Autodesk Fusion 360 part; units mm, degrees
(part 5 of 6)
sketch "Sketch6" plane through (0, -4, 0) normal (0, -1, 0) x (1, 0, 0)
  line L0 (159.495, -1.7823) -> (159.495, -3.7827)
  line L1 (159.495, -3.7827) -> (160.296, -3.7827)
  line L2 (160.296, -3.7827) -> (160.296, -6.8819)
  line L3 (160.296, -6.8819) -> (159.495, -6.8819)
  line L4 (159.495, -6.8819) -> (159.495, -12.6821)
  line L5 (159.495, -12.6821) -> (160.296, -12.6821)
  line L6 (160.296, -12.6821) -> (160.296, -15.7827)
  line L7 (160.296, -15.7827) -> (159.495, -15.7827)
  line L8 (159.495, -15.7827) -> (159.495, -17.7817)
  line L9 (159.495, -17.7817) -> (145.496, -17.7817)
  line L10 (145.496, -17.7817) -> (145.496, -15.7827)
  line L11 (145.496, -15.7827) -> (144.695, -15.7827)
  line L12 (144.695, -15.7827) -> (144.695, -12.6821)
  line L13 (144.695, -12.6821) -> (145.496, -12.6821)
  line L14 (145.496, -12.6821) -> (145.496, -6.8819)
  line L15 (145.496, -6.8819) -> (144.695, -6.8819)
  line L16 (144.695, -6.8819) -> (144.695, -3.7827)
  line L17 (144.695, -3.7827) -> (145.496, -3.7827)
  line L18 (145.496, -3.7827) -> (145.496, -1.7823)
  line L19 (145.496, -1.7823) -> (159.495, -1.7823)
  line L20 (31.196, -3.7827) -> (31.196, -1.7823)
  line L21 (31.196, -1.7823) -> (45.1954, -1.7823)
  line L22 (45.1954, -1.7823) -> (45.1954, -3.7827)
  line L23 (45.1954, -3.7827) -> (45.9962, -3.7827)
  line L24 (45.9962, -3.7827) -> (45.9962, -6.8819)
  line L25 (45.9962, -6.8819) -> (45.1954, -6.8819)
  line L26 (45.1954, -6.8819) -> (45.1954, -12.6821)
  line L27 (45.1954, -12.6821) -> (45.9962, -12.6821)
  line L28 (45.9962, -12.6821) -> (45.9962, -15.7827)
  line L29 (45.9962, -15.7827) -> (45.1954, -15.7827)
  line L30 (45.1954, -15.7827) -> (45.1954, -17.7817)
  line L31 (45.1954, -17.7817) -> (31.196, -17.7817)
  line L32 (31.196, -17.7817) -> (31.196, -15.7827)
  line L33 (31.196, -15.7827) -> (30.3954, -15.7827)
  line L34 (30.3954, -15.7827) -> (30.3954, -12.6821)
  line L35 (30.3954, -12.6821) -> (31.196, -12.6821)
  line L36 (31.196, -12.6821) -> (31.196, -6.8819)
  line L37 (31.196, -6.8819) -> (30.3954, -6.8819)
  line L38 (30.3954, -6.8819) -> (30.3954, -3.7827)
  line L39 (30.3954, -3.7827) -> (31.196, -3.7827)
  line L40 (155.021, -36.8316) -> (155.021, -34.8327)
  line L41 (155.021, -34.8327) -> (154.22, -34.8327)
  line L42 (154.22, -34.8327) -> (154.22, -31.7321)
  line L43 (154.22, -31.7321) -> (155.021, -31.7321)
  line L44 (155.021, -31.7321) -> (155.021, -25.9319)
  line L45 (155.021, -25.9319) -> (154.22, -25.9319)
  line L46 (154.22, -25.9319) -> (154.22, -22.8327)
  line L47 (154.22, -22.8327) -> (155.021, -22.8327)
  line L48 (155.021, -22.8327) -> (155.021, -20.8323)
  line L49 (155.021, -20.8323) -> (169.02, -20.8323)
  line L50 (169.02, -20.8323) -> (169.02, -22.8327)
  line L51 (169.02, -22.8327) -> (169.821, -22.8327)
  line L52 (169.821, -22.8327) -> (169.821, -25.9319)
  line L53 (169.821, -25.9319) -> (169.02, -25.9319)
  line L54 (169.02, -25.9319) -> (169.02, -31.7321)
  line L55 (169.02, -31.7321) -> (169.821, -31.7321)
  line L56 (169.821, -31.7321) -> (169.821, -34.8327)
  line L57 (169.821, -34.8327) -> (169.02, -34.8327)
  line L58 (169.02, -34.8327) -> (169.02, -36.8316)
  line L59 (169.02, -36.8316) -> (155.021, -36.8316)
  line L60 (135.971, -36.8316) -> (135.971, -34.8327)
  line L61 (135.971, -34.8327) -> (135.17, -34.8327)
  line L62 (135.17, -34.8327) -> (135.17, -31.7321)
  line L63 (135.17, -31.7321) -> (135.971, -31.7321)
  line L64 (135.971, -31.7321) -> (135.971, -25.9319)
  line L65 (135.971, -25.9319) -> (135.17, -25.9319)
  line L66 (135.17, -25.9319) -> (135.17, -22.8327)
  line L67 (135.17, -22.8327) -> (135.971, -22.8327)
  line L68 (135.971, -22.8327) -> (135.971, -20.8323)
  line L69 (135.971, -20.8323) -> (149.97, -20.8323)
  line L70 (149.97, -20.8323) -> (149.97, -22.8327)
  line L71 (149.97, -22.8327) -> (150.771, -22.8327)
  line L72 (150.771, -22.8327) -> (150.771, -25.9319)
  line L73 (150.771, -25.9319) -> (149.97, -25.9319)
  line L74 (149.97, -25.9319) -> (149.97, -31.7321)
  line L75 (149.97, -31.7321) -> (150.771, -31.7321)
  line L76 (150.771, -31.7321) -> (150.771, -34.8327)
  line L77 (150.771, -34.8327) -> (149.97, -34.8327)
  line L78 (149.97, -34.8327) -> (149.97, -36.8316)
  line L79 (149.97, -36.8316) -> (135.971, -36.8316)
  line L80 (116.92, -36.8316) -> (116.92, -34.8327)
  line L81 (116.92, -34.8327) -> (116.119, -34.8327)
  line L82 (116.119, -34.8327) -> (116.119, -31.7321)
  line L83 (116.119, -31.7321) -> (116.92, -31.7321)
  line L84 (116.92, -31.7321) -> (116.92, -25.9319)
  line L85 (116.92, -25.9319) -> (116.119, -25.9319)
  line L86 (116.119, -25.9319) -> (116.119, -22.8327)
  line L87 (116.119, -22.8327) -> (116.92, -22.8327)
  line L88 (116.92, -22.8327) -> (116.92, -20.8323)
  line L89 (116.92, -20.8323) -> (130.92, -20.8323)
  line L90 (130.92, -20.8323) -> (130.92, -22.8327)
  line L91 (130.92, -22.8327) -> (131.721, -22.8327)
  line L92 (131.721, -22.8327) -> (131.721, -25.9319)
  line L93 (131.721, -25.9319) -> (130.92, -25.9319)
  line L94 (130.92, -25.9319) -> (130.92, -31.7321)
  line L95 (130.92, -31.7321) -> (131.721, -31.7321)
  line L96 (131.721, -31.7321) -> (131.721, -34.8327)
  line L97 (131.721, -34.8327) -> (130.92, -34.8327)
  line L98 (130.92, -34.8327) -> (130.92, -36.8316)
  line L99 (130.92, -36.8316) -> (116.92, -36.8316)
  line L100 (111.869, -20.8323) -> (111.869, -22.8327)
  line L101 (111.869, -22.8327) -> (112.67, -22.8327)
  line L102 (112.67, -22.8327) -> (112.67, -25.9319)
  line L103 (112.67, -25.9319) -> (111.869, -25.9319)
  line L104 (111.869, -25.9319) -> (111.869, -31.7321)
  line L105 (111.869, -31.7321) -> (112.67, -31.7321)
  line L106 (112.67, -31.7321) -> (112.67, -34.8327)
  line L107 (112.67, -34.8327) -> (111.869, -34.8327)
  line L108 (111.869, -34.8327) -> (111.869, -36.8316)
  line L109 (111.869, -36.8316) -> (97.8697, -36.8316)
  line L110 (97.8697, -36.8316) -> (97.8697, -34.8327)
  line L111 (97.8697, -34.8327) -> (97.0703, -34.8327)
  line L112 (97.0703, -34.8327) -> (97.0703, -31.7321)
  line L113 (97.0703, -31.7321) -> (97.8697, -31.7321)
  line L114 (97.8697, -31.7321) -> (97.8697, -25.9319)
  line L115 (97.8697, -25.9319) -> (97.0703, -25.9319)
  line L116 (97.0703, -25.9319) -> (97.0703, -22.8327)
  line L117 (97.0703, -22.8327) -> (97.8697, -22.8327)
  line L118 (97.8697, -22.8327) -> (97.8697, -20.8323)
  line L119 (97.8697, -20.8323) -> (111.869, -20.8323)
  line L120 (40.7211, -36.8316) -> (40.7211, -34.8327)
  line L121 (40.7211, -34.8327) -> (39.9203, -34.8327)
  line L122 (39.9203, -34.8327) -> (39.9203, -31.7321)
  line L123 (39.9203, -31.7321) -> (40.7211, -31.7321)
  line L124 (40.7211, -31.7321) -> (40.7211, -25.9319)
  line L125 (40.7211, -25.9319) -> (39.9203, -25.9319)
  line L126 (39.9203, -25.9319) -> (39.9203, -22.8327)
  line L127 (39.9203, -22.8327) -> (40.7211, -22.8327)
  line L128 (40.7211, -22.8327) -> (40.7211, -20.8323)
  line L129 (40.7211, -20.8323) -> (54.7204, -20.8323)
  line L130 (54.7204, -20.8323) -> (54.7204, -22.8327)
  line L131 (54.7204, -22.8327) -> (55.5212, -22.8327)
  line L132 (55.5212, -22.8327) -> (55.5212, -25.9319)
  line L133 (55.5212, -25.9319) -> (54.7204, -25.9319)
  line L134 (54.7204, -25.9319) -> (54.7204, -31.7321)
  line L135 (54.7204, -31.7321) -> (55.5212, -31.7321)
  line L136 (55.5212, -31.7321) -> (55.5212, -34.8327)
  line L137 (55.5212, -34.8327) -> (54.7204, -34.8327)
  line L138 (54.7204, -34.8327) -> (54.7204, -36.8316)
  line L139 (54.7204, -36.8316) -> (40.7211, -36.8316)
  line L140 (35.6704, -20.8323) -> (35.6704, -22.8327)
  line L141 (35.6704, -22.8327) -> (36.4712, -22.8327)
  line L142 (36.4712, -22.8327) -> (36.4712, -25.9319)
  line L143 (36.4712, -25.9319) -> (35.6704, -25.9319)
  line L144 (35.6704, -25.9319) -> (35.6704, -31.7321)
  line L145 (35.6704, -31.7321) -> (36.4712, -31.7321)
  line L146 (36.4712, -31.7321) -> (36.4712, -34.8327)
  line L147 (36.4712, -34.8327) -> (35.6704, -34.8327)
  line L148 (35.6704, -34.8327) -> (35.6704, -36.8316)
  line L149 (35.6704, -36.8316) -> (21.671, -36.8316)
  line L150 (21.671, -36.8316) -> (21.671, -34.8327)
  line L151 (21.671, -34.8327) -> (20.8704, -34.8327)
  line L152 (20.8704, -34.8327) -> (20.8704, -31.7321)
  line L153 (20.8704, -31.7321) -> (21.671, -31.7321)
  line L154 (21.671, -31.7321) -> (21.671, -25.9319)
  line L155 (21.671, -25.9319) -> (20.8704, -25.9319)
  line L156 (20.8704, -25.9319) -> (20.8704, -22.8327)
  line L157 (20.8704, -22.8327) -> (21.671, -22.8327)
  line L158 (21.671, -22.8327) -> (21.671, -20.8323)
  line L159 (21.671, -20.8323) -> (35.6704, -20.8323)
  line L160 (155.021, -55.8816) -> (155.021, -53.8826)
  line L161 (155.021, -53.8826) -> (154.22, -53.8826)
  line L162 (154.22, -53.8826) -> (154.22, -50.782)
  line L163 (154.22, -50.782) -> (155.021, -50.782)
  line L164 (155.021, -50.782) -> (155.021, -44.982)
  line L165 (155.021, -44.982) -> (154.22, -44.982)
  line L166 (154.22, -44.982) -> (154.22, -41.8828)
  line L167 (154.22, -41.8828) -> (155.021, -41.8828)
  line L168 (155.021, -41.8828) -> (155.021, -39.8824)
  line L169 (155.021, -39.8824) -> (169.02, -39.8824)
  line L170 (169.02, -39.8824) -> (169.02, -41.8828)
  line L171 (169.02, -41.8828) -> (169.821, -41.8828)
  line L172 (169.821, -41.8828) -> (169.821, -44.982)
  line L173 (169.821, -44.982) -> (169.02, -44.982)
  line L174 (169.02, -44.982) -> (169.02, -50.782)
  line L175 (169.02, -50.782) -> (169.821, -50.782)
  line L176 (169.821, -50.782) -> (169.821, -53.8826)
  line L177 (169.821, -53.8826) -> (169.02, -53.8826)
  line L178 (169.02, -53.8826) -> (169.02, -55.8816)
  line L179 (169.02, -55.8816) -> (155.021, -55.8816)
  line L180 (16.6205, -20.8323) -> (16.6205, -22.8327)
  line L181 (16.6205, -22.8327) -> (17.4212, -22.8327)
  line L182 (17.4212, -22.8327) -> (17.4212, -25.9319)
  line L183 (17.4212, -25.9319) -> (16.6205, -25.9319)
  line L184 (16.6205, -25.9319) -> (16.6205, -31.7321)
  line L185 (16.6205, -31.7321) -> (17.4212, -31.7321)
  line L186 (17.4212, -31.7321) -> (17.4212, -34.8327)
  line L187 (17.4212, -34.8327) -> (16.6205, -34.8327)
  line L188 (16.6205, -34.8327) -> (16.6205, -36.8316)
  line L189 (16.6205, -36.8316) -> (2.621, -36.8316)
  line L190 (2.621, -36.8316) -> (2.621, -34.8327)
  line L191 (2.621, -34.8327) -> (1.8204, -34.8327)
  line L192 (1.8204, -34.8327) -> (1.8204, -31.7321)
  line L193 (1.8204, -31.7321) -> (2.621, -31.7321)
  line L194 (2.621, -31.7321) -> (2.621, -25.9319)
  line L195 (2.621, -25.9319) -> (1.8204, -25.9319)
  line L196 (1.8204, -25.9319) -> (1.8204, -22.8327)
  line L197 (1.8204, -22.8327) -> (2.621, -22.8327)
  line L198 (2.621, -22.8327) -> (2.621, -20.8323)
  line L199 (2.621, -20.8323) -> (16.6205, -20.8323)
  line L200 (21.671, -55.8816) -> (21.671, -53.8826)
  line L201 (21.671, -53.8826) -> (20.8704, -53.8826)
  line L202 (20.8704, -53.8826) -> (20.8704, -50.782)
  line L203 (20.8704, -50.782) -> (21.671, -50.782)
  line L204 (21.671, -50.782) -> (21.671, -44.982)
  line L205 (21.671, -44.982) -> (20.8704, -44.982)
  line L206 (20.8704, -44.982) -> (20.8704, -41.8828)
  line L207 (20.8704, -41.8828) -> (21.671, -41.8828)
  line L208 (21.671, -41.8828) -> (21.671, -39.8824)
  line L209 (21.671, -39.8824) -> (35.6704, -39.8824)
  line L210 (35.6704, -39.8824) -> (35.6704, -41.8828)
  line L211 (35.6704, -41.8828) -> (36.4712, -41.8828)
  line L212 (36.4712, -41.8828) -> (36.4712, -44.982)
  line L213 (36.4712, -44.982) -> (35.6704, -44.982)
  line L214 (35.6704, -44.982) -> (35.6704, -50.782)
  line L215 (35.6704, -50.782) -> (36.4712, -50.782)
  line L216 (36.4712, -50.782) -> (36.4712, -53.8826)
  line L217 (36.4712, -53.8826) -> (35.6704, -53.8826)
  line L218 (35.6704, -53.8826) -> (35.6704, -55.8816)
  line L219 (35.6704, -55.8816) -> (21.671, -55.8816)
  line L220 (97.8697, -55.8816) -> (97.8697, -53.8826)
  line L221 (97.8697, -53.8826) -> (97.0703, -53.8826)
  line L222 (97.0703, -53.8826) -> (97.0703, -50.782)
  line L223 (97.0703, -50.782) -> (97.8697, -50.782)
  line L224 (97.8697, -50.782) -> (97.8697, -44.982)
  line L225 (97.8697, -44.982) -> (97.0703, -44.982)
  line L226 (97.0703, -44.982) -> (97.0703, -41.8828)
  line L227 (97.0703, -41.8828) -> (97.8697, -41.8828)
  line L228 (97.8697, -41.8828) -> (97.8697, -39.8824)
  line L229 (97.8697, -39.8824) -> (111.869, -39.8824)
  line L230 (111.869, -39.8824) -> (111.869, -41.8828)
  line L231 (111.869, -41.8828) -> (112.67, -41.8828)
  line L232 (112.67, -41.8828) -> (112.67, -44.982)
  line L233 (112.67, -44.982) -> (111.869, -44.982)
  line L234 (111.869, -44.982) -> (111.869, -50.782)
  line L235 (111.869, -50.782) -> (112.67, -50.782)
  line L236 (112.67, -50.782) -> (112.67, -53.8826)
  line L237 (112.67, -53.8826) -> (111.869, -53.8826)
  line L238 (111.869, -53.8826) -> (111.869, -55.8816)
  line L239 (111.869, -55.8816) -> (97.8697, -55.8816)
  line L240 (54.7204, -39.8824) -> (54.7204, -41.8828)
  line L241 (54.7204, -41.8828) -> (55.5212, -41.8828)
  line L242 (55.5212, -41.8828) -> (55.5212, -44.982)
  line L243 (55.5212, -44.982) -> (54.7204, -44.982)
  line L244 (54.7204, -44.982) -> (54.7204, -50.782)
  line L245 (54.7204, -50.782) -> (55.5212, -50.782)
  line L246 (55.5212, -50.782) -> (55.5212, -53.8826)
  line L247 (55.5212, -53.8826) -> (54.7204, -53.8826)
  line L248 (54.7204, -53.8826) -> (54.7204, -55.8816)
  line L249 (54.7204, -55.8816) -> (40.7211, -55.8816)
  line L250 (40.7211, -55.8816) -> (40.7211, -53.8826)
  line L251 (40.7211, -53.8826) -> (39.9203, -53.8826)
  line L252 (39.9203, -53.8826) -> (39.9203, -50.782)
  line L253 (39.9203, -50.782) -> (40.7211, -50.782)
  line L254 (40.7211, -50.782) -> (40.7211, -44.982)
  line L255 (40.7211, -44.982) -> (39.9203, -44.982)
  line L256 (39.9203, -44.982) -> (39.9203, -41.8828)
  line L257 (39.9203, -41.8828) -> (40.7211, -41.8828)
  line L258 (40.7211, -41.8828) -> (40.7211, -39.8824)
  line L259 (40.7211, -39.8824) -> (54.7204, -39.8824)
  line L260 (92.8204, -20.8323) -> (92.8204, -22.8327)
  line L261 (92.8204, -22.8327) -> (93.6198, -22.8327)
  line L262 (93.6198, -22.8327) -> (93.6198, -25.9319)
  line L263 (93.6198, -25.9319) -> (92.8204, -25.9319)
  line L264 (92.8204, -25.9319) -> (92.8204, -31.7321)
  line L265 (92.8204, -31.7321) -> (93.6198, -31.7321)
  line L266 (93.6198, -31.7321) -> (93.6198, -34.8327)
  line L267 (93.6198, -34.8327) -> (92.8204, -34.8327)
  line L268 (92.8204, -34.8327) -> (92.8204, -36.8316)
  line L269 (92.8204, -36.8316) -> (78.8211, -36.8316)
  line L270 (78.8211, -36.8316) -> (78.8211, -34.8327)
  line L271 (78.8211, -34.8327) -> (78.0203, -34.8327)
  line L272 (78.0203, -34.8327) -> (78.0203, -31.7321)
  line L273 (78.0203, -31.7321) -> (78.8211, -31.7321)
  line L274 (78.8211, -31.7321) -> (78.8211, -25.9319)
  line L275 (78.8211, -25.9319) -> (78.0203, -25.9319)
  line L276 (78.0203, -25.9319) -> (78.0203, -22.8327)
  line L277 (78.0203, -22.8327) -> (78.8211, -22.8327)
  line L278 (78.8211, -22.8327) -> (78.8211, -20.8323)
  line L279 (78.8211, -20.8323) -> (92.8204, -20.8323)
  line L280 (130.92, -39.8824) -> (130.92, -41.8828)
  line L281 (130.92, -41.8828) -> (131.721, -41.8828)
  line L282 (131.721, -41.8828) -> (131.721, -44.982)
  line L283 (131.721, -44.982) -> (130.92, -44.982)
  line L284 (130.92, -44.982) -> (130.92, -50.782)
  line L285 (130.92, -50.782) -> (131.721, -50.782)
  line L286 (131.721, -50.782) -> (131.721, -53.8826)
  line L287 (131.721, -53.8826) -> (130.92, -53.8826)
  line L288 (130.92, -53.8826) -> (130.92, -55.8816)
  line L289 (130.92, -55.8816) -> (116.92, -55.8816)
  line L290 (116.92, -55.8816) -> (116.92, -53.8826)
  line L291 (116.92, -53.8826) -> (116.119, -53.8826)
  line L292 (116.119, -53.8826) -> (116.119, -50.782)
  line L293 (116.119, -50.782) -> (116.92, -50.782)
  line L294 (116.92, -50.782) -> (116.92, -44.982)
  line L295 (116.92, -44.982) -> (116.119, -44.982)
  line L296 (116.119, -44.982) -> (116.119, -41.8828)
  line L297 (116.119, -41.8828) -> (116.92, -41.8828)
  line L298 (116.92, -41.8828) -> (116.92, -39.8824)
  line L299 (116.92, -39.8824) -> (130.92, -39.8824)
  line L300 (188.07, -20.8323) -> (188.07, -22.8327)
  line L301 (188.07, -22.8327) -> (188.871, -22.8327)
  line L302 (188.871, -22.8327) -> (188.871, -25.9319)
  line L303 (188.871, -25.9319) -> (188.07, -25.9319)
  line L304 (188.07, -25.9319) -> (188.07, -31.7321)
  line L305 (188.07, -31.7321) -> (188.871, -31.7321)
  line L306 (188.871, -31.7321) -> (188.871, -34.8327)
  line L307 (188.871, -34.8327) -> (188.07, -34.8327)
  line L308 (188.07, -34.8327) -> (188.07, -36.8316)
  line L309 (188.07, -36.8316) -> (174.071, -36.8316)
  line L310 (174.071, -36.8316) -> (174.071, -34.8327)
  line L311 (174.071, -34.8327) -> (173.27, -34.8327)
  line L312 (173.27, -34.8327) -> (173.27, -31.7321)
  line L313 (173.27, -31.7321) -> (174.071, -31.7321)
  line L314 (174.071, -31.7321) -> (174.071, -25.9319)
  line L315 (174.071, -25.9319) -> (173.27, -25.9319)
  line L316 (173.27, -25.9319) -> (173.27, -22.8327)
  line L317 (173.27, -22.8327) -> (174.071, -22.8327)
  line L318 (174.071, -22.8327) -> (174.071, -20.8323)
  line L319 (174.071, -20.8323) -> (188.07, -20.8323)
  line L320 (69.2961, -17.7817) -> (69.2961, -15.7827)
  line L321 (69.2961, -15.7827) -> (68.4953, -15.7827)
  line L322 (68.4953, -15.7827) -> (68.4953, -12.6821)
  line L323 (68.4953, -12.6821) -> (69.2961, -12.6821)
  line L324 (69.2961, -12.6821) -> (69.2961, -6.8819)
  line L325 (69.2961, -6.8819) -> (68.4953, -6.8819)
  line L326 (68.4953, -6.8819) -> (68.4953, -3.7827)
  line L327 (68.4953, -3.7827) -> (69.2961, -3.7827)
  line L328 (69.2961, -3.7827) -> (69.2961, -1.7823)
  line L329 (69.2961, -1.7823) -> (83.2954, -1.7823)
  line L330 (83.2954, -1.7823) -> (83.2954, -3.7827)
  line L331 (83.2954, -3.7827) -> (84.0962, -3.7827)
  line L332 (84.0962, -3.7827) -> (84.0962, -6.8819)
  line L333 (84.0962, -6.8819) -> (83.2954, -6.8819)
  line L334 (83.2954, -6.8819) -> (83.2954, -12.6821)
  line L335 (83.2954, -12.6821) -> (84.0962, -12.6821)
  line L336 (84.0962, -12.6821) -> (84.0962, -15.7827)
  line L337 (84.0962, -15.7827) -> (83.2954, -15.7827)
  line L338 (83.2954, -15.7827) -> (83.2954, -17.7817)
  line L339 (83.2954, -17.7817) -> (69.2961, -17.7817)
  line L340 (164.546, -17.7817) -> (164.546, -15.7827)
  line L341 (164.546, -15.7827) -> (163.745, -15.7827)
  line L342 (163.745, -15.7827) -> (163.745, -12.6821)
  line L343 (163.745, -12.6821) -> (164.546, -12.6821)
  line L344 (164.546, -12.6821) -> (164.546, -6.8819)
  line L345 (164.546, -6.8819) -> (163.745, -6.8819)
  line L346 (163.745, -6.8819) -> (163.745, -3.7827)
  line L347 (163.745, -3.7827) -> (164.546, -3.7827)
  line L348 (164.546, -3.7827) -> (164.546, -1.7823)
  line L349 (164.546, -1.7823) -> (178.545, -1.7823)
  line L350 (178.545, -1.7823) -> (178.545, -3.7827)
  line L351 (178.545, -3.7827) -> (179.346, -3.7827)
  line L352 (179.346, -3.7827) -> (179.346, -6.8819)
  line L353 (179.346, -6.8819) -> (178.545, -6.8819)
  line L354 (178.545, -6.8819) -> (178.545, -12.6821)
  line L355 (178.545, -12.6821) -> (179.346, -12.6821)
  line L356 (179.346, -12.6821) -> (179.346, -15.7827)
  line L357 (179.346, -15.7827) -> (178.545, -15.7827)
  line L358 (178.545, -15.7827) -> (178.545, -17.7817)
  line L359 (178.545, -17.7817) -> (164.546, -17.7817)
  line L360 (64.2454, -1.7823) -> (64.2454, -3.7827)
  line L361 (64.2454, -3.7827) -> (65.0462, -3.7827)
  line L362 (65.0462, -3.7827) -> (65.0462, -6.8819)
  line L363 (65.0462, -6.8819) -> (64.2454, -6.8819)
  line L364 (64.2454, -6.8819) -> (64.2454, -12.6821)
  line L365 (64.2454, -12.6821) -> (65.0462, -12.6821)
  line L366 (65.0462, -12.6821) -> (65.0462, -15.7827)
  line L367 (65.0462, -15.7827) -> (64.2454, -15.7827)
  line L368 (64.2454, -15.7827) -> (64.2454, -17.7817)
  line L369 (64.2454, -17.7817) -> (50.2461, -17.7817)
  line L370 (50.2461, -17.7817) -> (50.2461, -15.7827)
  line L371 (50.2461, -15.7827) -> (49.4453, -15.7827)
  line L372 (49.4453, -15.7827) -> (49.4453, -12.6821)
  line L373 (49.4453, -12.6821) -> (50.2461, -12.6821)
  line L374 (50.2461, -12.6821) -> (50.2461, -6.8819)
  line L375 (50.2461, -6.8819) -> (49.4453, -6.8819)
  line L376 (49.4453, -6.8819) -> (49.4453, -3.7827)
  line L377 (49.4453, -3.7827) -> (50.2461, -3.7827)
  line L378 (50.2461, -3.7827) -> (50.2461, -1.7823)
  line L379 (50.2461, -1.7823) -> (64.2454, -1.7823)
  line L380 (126.446, -3.7827) -> (126.446, -1.7823)
  line L381 (126.446, -1.7823) -> (140.445, -1.7823)
  line L382 (140.445, -1.7823) -> (140.445, -3.7827)
  line L383 (140.445, -3.7827) -> (141.246, -3.7827)
  line L384 (141.246, -3.7827) -> (141.246, -6.8819)
  line L385 (141.246, -6.8819) -> (140.445, -6.8819)
  line L386 (140.445, -6.8819) -> (140.445, -12.6821)
  line L387 (140.445, -12.6821) -> (141.246, -12.6821)
  line L388 (141.246, -12.6821) -> (141.246, -15.7827)
  line L389 (141.246, -15.7827) -> (140.445, -15.7827)
  line L390 (140.445, -15.7827) -> (140.445, -17.7817)
  line L391 (140.445, -17.7817) -> (126.446, -17.7817)
  line L392 (126.446, -17.7817) -> (126.446, -15.7827)
  line L393 (126.446, -15.7827) -> (125.645, -15.7827)
  line L394 (125.645, -15.7827) -> (125.645, -12.6821)
  line L395 (125.645, -12.6821) -> (126.446, -12.6821)
  line L396 (126.446, -12.6821) -> (126.446, -6.8819)
  line L397 (126.446, -6.8819) -> (125.645, -6.8819)
  line L398 (125.645, -6.8819) -> (125.645, -3.7827)
  line L399 (125.645, -3.7827) -> (126.446, -3.7827)
  line L400 (92.8204, -53.8826) -> (92.8204, -55.8816)
  line L401 (92.8204, -55.8816) -> (78.8211, -55.8816)
  line L402 (78.8211, -55.8816) -> (78.8211, -53.8826)
  line L403 (78.8211, -53.8826) -> (78.0203, -53.8826)
  line L404 (78.0203, -53.8826) -> (78.0203, -50.782)
  line L405 (78.0203, -50.782) -> (78.8211, -50.782)
  line L406 (78.8211, -50.782) -> (78.8211, -44.982)
  line L407 (78.8211, -44.982) -> (78.0203, -44.982)
  line L408 (78.0203, -44.982) -> (78.0203, -41.8828)
  line L409 (78.0203, -41.8828) -> (78.8211, -41.8828)
  line L410 (78.8211, -41.8828) -> (78.8211, -39.8824)
  line L411 (78.8211, -39.8824) -> (92.8204, -39.8824)
  line L412 (92.8204, -39.8824) -> (92.8204, -41.8828)
  line L413 (92.8204, -41.8828) -> (93.6198, -41.8828)
  line L414 (93.6198, -41.8828) -> (93.6198, -44.982)
  line L415 (93.6198, -44.982) -> (92.8204, -44.982)
  line L416 (92.8204, -44.982) -> (92.8204, -50.782)
  line L417 (92.8204, -50.782) -> (93.6198, -50.782)
  line L418 (93.6198, -50.782) -> (93.6198, -53.8826)
  line L419 (93.6198, -53.8826) -> (92.8204, -53.8826)
  line L420 (135.971, -41.8828) -> (135.971, -39.8824)
  line L421 (135.971, -39.8824) -> (149.97, -39.8824)
  line L422 (149.97, -39.8824) -> (149.97, -41.8828)
  line L423 (149.97, -41.8828) -> (150.771, -41.8828)
  line L424 (150.771, -41.8828) -> (150.771, -44.982)
  line L425 (150.771, -44.982) -> (149.97, -44.982)
  line L426 (149.97, -44.982) -> (149.97, -50.782)
  line L427 (149.97, -50.782) -> (150.771, -50.782)
  line L428 (150.771, -50.782) -> (150.771, -53.8826)
  line L429 (150.771, -53.8826) -> (149.97, -53.8826)
  line L430 (149.97, -53.8826) -> (149.97, -55.8816)
  line L431 (149.97, -55.8816) -> (135.971, -55.8816)
  line L432 (135.971, -55.8816) -> (135.971, -53.8826)
  line L433 (135.971, -53.8826) -> (135.17, -53.8826)
  line L434 (135.17, -53.8826) -> (135.17, -50.782)
  line L435 (135.17, -50.782) -> (135.971, -50.782)
  line L436 (135.971, -50.782) -> (135.971, -44.982)
  line L437 (135.971, -44.982) -> (135.17, -44.982)
  line L438 (135.17, -44.982) -> (135.17, -41.8828)
  line L439 (135.17, -41.8828) -> (135.971, -41.8828)
  line L440 (59.7711, -41.8828) -> (59.7711, -39.8824)
  line L441 (59.7711, -39.8824) -> (73.7704, -39.8824)
  line L442 (73.7704, -39.8824) -> (73.7704, -41.8828)
  line L443 (73.7704, -41.8828) -> (74.5712, -41.8828)
  line L444 (74.5712, -41.8828) -> (74.5712, -44.982)
  line L445 (74.5712, -44.982) -> (73.7704, -44.982)
  line L446 (73.7704, -44.982) -> (73.7704, -50.782)
  line L447 (73.7704, -50.782) -> (74.5712, -50.782)
  line L448 (74.5712, -50.782) -> (74.5712, -53.8826)
  line L449 (74.5712, -53.8826) -> (73.7704, -53.8826)
  line L450 (73.7704, -53.8826) -> (73.7704, -55.8816)
  line L451 (73.7704, -55.8816) -> (59.7711, -55.8816)
  line L452 (59.7711, -55.8816) -> (59.7711, -53.8826)
  line L453 (59.7711, -53.8826) -> (58.9703, -53.8826)
  line L454 (58.9703, -53.8826) -> (58.9703, -50.782)
  line L455 (58.9703, -50.782) -> (59.7711, -50.782)
  line L456 (59.7711, -50.782) -> (59.7711, -44.982)
  line L457 (59.7711, -44.982) -> (58.9703, -44.982)
  line L458 (58.9703, -44.982) -> (58.9703, -41.8828)
  line L459 (58.9703, -41.8828) -> (59.7711, -41.8828)
  line L460 (16.6205, -53.8826) -> (16.6205, -55.8816)
  line L461 (16.6205, -55.8816) -> (2.621, -55.8816)
  line L462 (2.621, -55.8816) -> (2.621, -53.8826)
  line L463 (2.621, -53.8826) -> (1.8204, -53.8826)
  line L464 (1.8204, -53.8826) -> (1.8204, -50.782)
  line L465 (1.8204, -50.782) -> (2.621, -50.782)
  line L466 (2.621, -50.782) -> (2.621, -44.982)
  line L467 (2.621, -44.982) -> (1.8204, -44.982)
  line L468 (1.8204, -44.982) -> (1.8204, -41.8828)
  line L469 (1.8204, -41.8828) -> (2.621, -41.8828)
  line L470 (2.621, -41.8828) -> (2.621, -39.8824)
  line L471 (2.621, -39.8824) -> (16.6205, -39.8824)
  line L472 (16.6205, -39.8824) -> (16.6205, -41.8828)
  line L473 (16.6205, -41.8828) -> (17.4212, -41.8828)
  line L474 (17.4212, -41.8828) -> (17.4212, -44.982)
  line L475 (17.4212, -44.982) -> (16.6205, -44.982)
  line L476 (16.6205, -44.982) -> (16.6205, -50.782)
  line L477 (16.6205, -50.782) -> (17.4212, -50.782)
  line L478 (17.4212, -50.782) -> (17.4212, -53.8826)
  line L479 (17.4212, -53.8826) -> (16.6205, -53.8826)
  line L480 (174.071, -41.8828) -> (174.071, -39.8824)
  line L481 (174.071, -39.8824) -> (188.07, -39.8824)
  line L482 (188.07, -39.8824) -> (188.07, -41.8828)
  line L483 (188.07, -41.8828) -> (188.871, -41.8828)
  line L484 (188.871, -41.8828) -> (188.871, -44.982)
  line L485 (188.871, -44.982) -> (188.07, -44.982)
  line L486 (188.07, -44.982) -> (188.07, -50.782)
  line L487 (188.07, -50.782) -> (188.871, -50.782)
  line L488 (188.871, -50.782) -> (188.871, -53.8826)
  line L489 (188.871, -53.8826) -> (188.07, -53.8826)
  line L490 (188.07, -53.8826) -> (188.07, -55.8816)
  line L491 (188.07, -55.8816) -> (174.071, -55.8816)
  line L492 (174.071, -55.8816) -> (174.071, -53.8826)
  line L493 (174.071, -53.8826) -> (173.27, -53.8826)
  line L494 (173.27, -53.8826) -> (173.27, -50.782)
  line L495 (173.27, -50.782) -> (174.071, -50.782)
  line L496 (174.071, -50.782) -> (174.071, -44.982)
  line L497 (174.071, -44.982) -> (173.27, -44.982)
  line L498 (173.27, -44.982) -> (173.27, -41.8828)
  line L499 (173.27, -41.8828) -> (174.071, -41.8828)
  line L500 (73.7704, -34.8327) -> (73.7704, -36.8316)
  line L501 (73.7704, -36.8316) -> (59.7711, -36.8316)
  line L502 (59.7711, -36.8316) -> (59.7711, -34.8327)
  line L503 (59.7711, -34.8327) -> (58.9703, -34.8327)
  line L504 (58.9703, -34.8327) -> (58.9703, -31.7321)
  line L505 (58.9703, -31.7321) -> (59.7711, -31.7321)
  line L506 (59.7711, -31.7321) -> (59.7711, -25.9319)
  line L507 (59.7711, -25.9319) -> (58.9703, -25.9319)
  line L508 (58.9703, -25.9319) -> (58.9703, -22.8327)
  line L509 (58.9703, -22.8327) -> (59.7711, -22.8327)
  line L510 (59.7711, -22.8327) -> (59.7711, -20.8323)
  line L511 (59.7711, -20.8323) -> (73.7704, -20.8323)
  line L512 (73.7704, -20.8323) -> (73.7704, -22.8327)
  line L513 (73.7704, -22.8327) -> (74.5712, -22.8327)
  line L514 (74.5712, -22.8327) -> (74.5712, -25.9319)
  line L515 (74.5712, -25.9319) -> (73.7704, -25.9319)
  line L516 (73.7704, -25.9319) -> (73.7704, -31.7321)
  line L517 (73.7704, -31.7321) -> (74.5712, -31.7321)
  line L518 (74.5712, -31.7321) -> (74.5712, -34.8327)
  line L519 (74.5712, -34.8327) -> (73.7704, -34.8327)
  line L520 (26.1455, -15.7827) -> (26.1455, -17.7817)
  line L521 (26.1455, -17.7817) -> (12.146, -17.7817)
  line L522 (12.146, -17.7817) -> (12.146, -15.7827)
  line L523 (12.146, -15.7827) -> (11.3454, -15.7827)
  line L524 (11.3454, -15.7827) -> (11.3454, -12.6821)
  line L525 (11.3454, -12.6821) -> (12.146, -12.6821)
  line L526 (12.146, -12.6821) -> (12.146, -6.8819)
  line L527 (12.146, -6.8819) -> (11.3454, -6.8819)
  line L528 (11.3454, -6.8819) -> (11.3454, -3.7827)
  line L529 (11.3454, -3.7827) -> (12.146, -3.7827)
  line L530 (12.146, -3.7827) -> (12.146, -1.7823)
  line L531 (12.146, -1.7823) -> (26.1455, -1.7823)
  line L532 (26.1455, -1.7823) -> (26.1455, -3.7827)
  line L533 (26.1455, -3.7827) -> (26.9462, -3.7827)
  line L534 (26.9462, -3.7827) -> (26.9462, -6.8819)
  line L535 (26.9462, -6.8819) -> (26.1455, -6.8819)
  line L536 (26.1455, -6.8819) -> (26.1455, -12.6821)
  line L537 (26.1455, -12.6821) -> (26.9462, -12.6821)
  line L538 (26.9462, -12.6821) -> (26.9462, -15.7827)
  line L539 (26.9462, -15.7827) -> (26.1455, -15.7827)
  arc A0 (190.596, -18.7817) -> (188.596, -16.7817) centre (188.596, -18.7817) ccw
  line L540 (188.596, -16.7817) -> (184.846, -16.7817)
  arc A1 (182.846, -14.7817) -> (184.846, -16.7817) centre (184.846, -14.7817) ccw
  line L541 (182.846, -14.7817) -> (182.846, -2.2564)
  arc A2 (182.846, -2.2564) -> (180.846, -0.2564) centre (180.846, -2.2564) ccw
  line L542 (180.846, -0.2564) -> (167.0351, -0.2565)
  arc A3 (9.8454, -0.2576) -> (7.8454, -2.2576) centre (9.8454, -2.2576) ccw
  line L543 (7.8454, -2.2576) -> (7.8454, -14.7817)
  arc A4 (5.8454, -16.7817) -> (7.8454, -14.7817) centre (5.8454, -14.7817) ccw
  line L544 (5.8454, -16.7817) -> (2.0951, -16.7817)
  arc A5 (2.0951, -16.7817) -> (0.0951, -18.7817) centre (2.0951, -18.7817) ccw
  line L545 (0.0951, -18.7817) -> (0.0951, -55.4069)
  line L546 (0.0951, -55.4069) -> (0.102, -55.5639)
  line L547 (0.102, -55.5639) -> (0.1199, -55.7209)
  line L548 (0.1199, -55.7209) -> (0.1502, -55.874)
  line L549 (0.1502, -55.874) -> (0.1929, -56.0268)
  line L550 (0.1929, -56.0268) -> (0.248, -56.1728)
  line L551 (0.248, -56.1728) -> (0.3128, -56.315)
  line L552 (0.3128, -56.315) -> (0.39, -56.4526)
  line L553 (0.39, -56.4526) -> (0.4768, -56.5838)
  line L554 (0.4768, -56.5838) -> (0.5746, -56.7062)
  line L555 (0.5746, -56.7062) -> (0.6808, -56.8219)
  line L556 (0.6808, -56.8219) -> (0.7965, -56.9281)
  line L557 (0.7965, -56.9281) -> (0.9192, -57.0258)
  line L558 (0.9192, -57.0258) -> (1.0501, -57.113)
  line L559 (1.0501, -57.113) -> (1.1879, -57.1899)
  line L560 (1.1879, -57.1899) -> (1.3298, -57.2548)
  line L561 (1.3298, -57.2548) -> (1.4759, -57.3098)
  line L562 (1.4759, -57.3098) -> (1.6288, -57.3525)
  line L563 (1.6288, -57.3525) -> (1.7818, -57.3828)
  line L564 (1.7818, -57.3828) -> (1.9389, -57.4008)
  line L565 (1.9389, -57.4008) -> (2.096, -57.4075)
  line L566 (2.096, -57.4075) -> (6.5216, -57.4075)
  line L567 (188.597, -57.4075) -> (188.753, -57.4008)
  line L568 (188.753, -57.4008) -> (188.908, -57.3828)
  line L569 (188.908, -57.3828) -> (189.063, -57.3525)
  line L570 (189.063, -57.3525) -> (189.214, -57.3098)
  line L571 (189.214, -57.3098) -> (189.362, -57.2548)
  line L572 (189.362, -57.2548) -> (189.504, -57.1899)
  line L573 (189.504, -57.1899) -> (189.64, -57.113)
  line L574 (189.64, -57.113) -> (189.771, -57.0258)
  line L575 (189.771, -57.0258) -> (189.895, -56.9281)
  line L576 (189.895, -56.9281) -> (190.011, -56.8219)
  line L577 (190.011, -56.8219) -> (190.117, -56.7062)
  line L578 (190.117, -56.7062) -> (190.215, -56.5838)
  line L579 (190.215, -56.5838) -> (190.302, -56.4526)
  line L580 (190.302, -56.4526) -> (190.379, -56.315)
  line L581 (190.379, -56.315) -> (190.444, -56.1728)
  line L582 (190.444, -56.1728) -> (190.499, -56.0268)
  line L583 (190.499, -56.0268) -> (190.54, -55.874)
  line L584 (190.54, -55.874) -> (190.572, -55.7209)
  line L585 (190.572, -55.7209) -> (190.59, -55.5639)
  line L586 (190.59, -55.5639) -> (190.596, -55.4069)
  line L587 (190.596, -55.4069) -> (190.596, -18.7817)
  line L588 (97.8711, -16.7817) -> (88.7705, -16.7817)
  line L589 (88.7705, -16.7817) -> (88.7705, -2.0326)
  line L590 (88.7705, -2.0326) -> (97.8711, -2.0326)
  line L591 (97.8711, -2.0326) -> (97.8711, -1.7823)
  line L592 (97.8711, -1.7823) -> (111.87, -1.7823)
  line L593 (111.87, -1.7823) -> (111.87, -2.0326)
  line L594 (111.87, -2.0326) -> (120.971, -2.0326)
  line L595 (120.971, -2.0326) -> (120.971, -16.7817)
  line L596 (120.971, -16.7817) -> (111.87, -16.7817)
  line L597 (111.87, -16.7817) -> (111.87, -17.7817)
  line L598 (111.87, -17.7817) -> (97.8711, -17.7817)
  line L599 (97.8711, -17.7817) -> (97.8711, -16.7817)
  line L600 (88.7705, -16.7817) -> (120.971, -16.7817)
  line L601 (120.971, -16.7817) -> (120.971, -19.8875)
  line L602 (120.971, -19.8875) -> (88.7705, -19.8875)
  line L603 (88.7705, -19.8875) -> (88.7705, -16.7817)
  line L604 (167.0351, -0.2565) -> (137.8078, -0.2567)
  line L605 (6.5216, -57.4075) -> (35.7006, -57.4075)
  line L606 (35.7006, -57.4075) -> (154.9924, -57.4075)
  line L607 (154.9924, -57.4075) -> (184.1714, -57.4075)
  line L608 (184.1714, -57.4075) -> (188.597, -57.4075)
  line L609 (137.8078, -0.2567) -> (52.887, -0.2573)
  line L610 (52.887, -0.2573) -> (23.4739, -0.2575)
  line L611 (23.4739, -0.2575) -> (9.8454, -0.2576)
  constraint perpendicular L600 L601
  constraint parallel L600 L602
  constraint parallel L601 L603
  constraint coincident L595.end L596.start
  constraint perpendicular L595 L600
  constraint coincident L588.end L589.start
extrude "Extrude8" cut sketch "Sketch6" against normal blind 3 contours L588 L596 L597 L598 L599 L600 L601 L602 L603